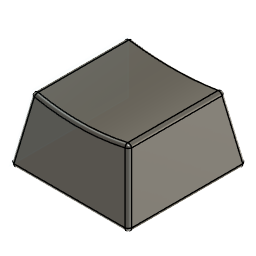
Keycap (Autodesk Fusion 360 design; units mm, degrees)
part number: 2026-06-10-19-01-09-596
Autodesk Fusion 360 part; units mm, degrees
sketch "Sketch1" plane through (0, 0, 0) normal (0, 0, 1) x (1, 0, 0)
  line L0 (9, 9) -> (-9, 9)
  line L1 (-9, 9) -> (-9, -9)
  line L2 (-9, -9) -> (9, -9)
  line L3 (9, -9) -> (9, 9)
  line L4 (9, 9) -> (-9, -9) construction
  line L5 (-9, 9) -> (9, -9) construction
  dimension "d1" = 18
  dimension "d2" = 18
  constraint horizontal L0
  constraint perpendicular L0 L1
  constraint parallel L0 L2
  constraint parallel L1 L3
  constraint coincident L4 origin
  constraint coincident L5 origin
  measures "d1" distance of L0.start L0.end
  measures "d2" distance of L0.start L2.end
extrude "Extrude1" add sketch "Sketch1" along normal blind 10 draft -10
sketch "Sketch2" plane through (-8.7286, 0, 1.5391) normal (-0.984808, 0, 0.173648) x (0, -1, 0)
  line L0 (7.2367, 8.5914) -> (-7.2367, 8.5914)
  line L1 (-7.2367, 8.5914) -> (-9, -1.5628)
  line L2 (-9, -1.5628) -> (9, -1.5628)
  line L3 (9, -1.5628) -> (7.2367, 8.5914)
sketch "Sketch3" plane through (0, 0, 0) normal (0, 1, 0) x (1, 0, 0)
  circle A0 centre (-0.4225, -45.9852) radius 36.7913
  point P0 (7.2367, -10)
  constraint coincident A0 P0
extrude "Extrude2" cut sketch "Sketch3" along normal mid plane 20
sketch "Sketch4" plane through (0, 0, 0) normal (0, 0, 1) x (1, 0, 0)
  line L0 (3, 0.35) -> (3, -0.35)
  line L1 (-3, -0.35) -> (-3, 0.35)
  line L2 (-3, 0.75) -> (3, -0.75) construction
  line L3 (3, 0.75) -> (-3, -0.75) construction
  line L4 (-0.35, 3) -> (0.35, 3)
  line L5 (0.35, -3) -> (-0.35, -3)
  line L6 (-0.75, 3) -> (0.75, -3) construction
  line L7 (0.75, 3) -> (-0.75, -3) construction
  line L8 (-0.75, -2.6) -> (-0.75, -1.15)
  line L9 (-0.75, 1.15) -> (-0.75, 2.6)
  line L10 (2.6, -0.75) -> (1.15, -0.75)
  line L11 (-1.15, -0.75) -> (-2.6, -0.75)
  line L12 (0.75, -1.15) -> (0.75, -2.6)
  line L13 (0.75, 2.6) -> (0.75, 1.15)
  line L14 (-2.6, 0.75) -> (-1.15, 0.75)
  line L15 (1.15, 0.75) -> (2.6, 0.75)
  arc A0 (-1.15, 0.75) -> (-0.75, 1.15) centre (-1.15, 1.15) ccw
  arc A1 (-2.6, 0.75) -> (-3, 0.35) centre (-2.6, 0.35) ccw
  arc A2 (-3, -0.35) -> (-2.6, -0.75) centre (-2.6, -0.35) ccw
  arc A3 (-0.75, -1.15) -> (-1.15, -0.75) centre (-1.15, -1.15) ccw
  arc A4 (-0.75, -2.6) -> (-0.35, -3) centre (-0.35, -2.6) ccw
  arc A5 (0.35, -3) -> (0.75, -2.6) centre (0.35, -2.6) ccw
  arc A6 (1.15, -0.75) -> (0.75, -1.15) centre (1.15, -1.15) ccw
  arc A7 (2.6, -0.75) -> (3, -0.35) centre (2.6, -0.35) ccw
  arc A8 (3, 0.35) -> (2.6, 0.75) centre (2.6, 0.35) ccw
  arc A9 (0.75, 1.15) -> (1.15, 0.75) centre (1.15, 1.15) ccw
  arc A10 (0.75, 2.6) -> (0.35, 3) centre (0.35, 2.6) ccw
  arc A11 (-0.35, 3) -> (-0.75, 2.6) centre (-0.35, 2.6) ccw
  dimension "d9" = 1.5
  dimension "d10" = 1.5
  dimension "d11" = 6
  dimension "d12" = 6
  dimension "d13" = 0.4
  dimension "d14" = 0.4
  dimension "d15" = 0.4
  dimension "d16" = 0.4
  dimension "d17" = 0.4
  dimension "d18" = 0.4
  dimension "d19" = 0.4
  dimension "d20" = 0.4
  dimension "d21" = 0.4
  dimension "d22" = 0.4
  dimension "d23" = 0.4
  dimension "d24" = 0.4
  constraint horizontal L14
  constraint perpendicular L0 L15
  constraint parallel L10 L15
  constraint parallel L0 L1
  constraint coincident L2 origin
  constraint coincident L3 origin
  constraint horizontal L4
  constraint perpendicular L4 L13
  constraint parallel L4 L5
  constraint parallel L8 L12
  constraint coincident L6 origin
  constraint coincident L7 origin
  constraint collinear L8 L9
  constraint collinear L10 L11
  constraint collinear L14 L15
  constraint tangent L9 A0
  constraint tangent L14 A0
  constraint coincident L2.start L14
  constraint coincident L2.start L1
  constraint tangent L14 A1
  constraint tangent L1 A1
  constraint coincident L3.end L11
  constraint coincident L3.end L1
  constraint tangent L11 A2
  constraint tangent L1 A2
  constraint tangent L8 A3
  constraint tangent L11 A3
  constraint coincident L7.end L5
  constraint coincident L7.end L8
  constraint tangent L5 A4
  constraint tangent L8 A4
  constraint coincident L6.end L5
  constraint coincident L6.end L12
  constraint tangent L5 A5
  constraint tangent L12 A5
  constraint tangent L10 A6
  constraint tangent L12 A6
  constraint coincident L2.end L10
  constraint coincident L2.end L0
  constraint tangent L10 A7
  constraint tangent L0 A7
  constraint coincident L3.start L0
  constraint coincident L3.start L15
  constraint tangent L0 A8
  constraint tangent L15 A8
  constraint tangent L15 A9
  constraint tangent L13 A9
  constraint coincident L7.start L13
  constraint coincident L7.start L4
  constraint tangent L13 A10
  constraint tangent L4 A10
  constraint coincident L6.start L4
  constraint coincident L6.start L9
  constraint tangent L4 A11
  constraint tangent L9 A11
  measures "d9" distance of L3.start L2.end
  measures "d10" distance of L6.end L7.end
  measures "d11" distance of L2.start L3.start
  measures "d12" distance of L6.start L7.end
  measures "d13" radius of A0
  measures "d14" radius of A1
  measures "d15" radius of A2
  measures "d16" radius of A3
  measures "d17" radius of A4
  measures "d18" radius of A5
  measures "d19" radius of A6
  measures "d20" radius of A7
  measures "d21" radius of A8
  measures "d22" radius of A9
  measures "d23" radius of A10
  measures "d24" radius of A11
extrude "Extrude3" cut sketch "Sketch4" along normal blind 8
fillet "Fillet2" radius 0.5 60 edges at (-7.2657, 0, 9.8359) (-9, 0, 0) (8.1184, 8.1184, 5) (8.1184, -8.1184, 5) (-8.1328, 8.1328, 4.918) (1.875, 0.75, 0) (0.8672, 0.8672, 0) (0.75, 1.875, 0) (0.6328, 2.8828, 0) (0, 3, 0) (-0.6328, 2.8828, 0) (-0.75, 1.875, 0) (-0.8672, 0.8672, 0) (-1.875, 0.75, 0) (-2.8828, 0.6328, 0) (-3, 0, 0) (-2.8828, -0.6328, 0) (-1.875, -0.75, 0) (-0.8672, -0.8672, 0) (-0.75, -1.875, 0) (-0.6328, -2.8828, 0) (0, -3, 0) (0.6328, -2.8828, 0) (0.75, -1.875, 0) (0.8672, -0.8672, 0) (1.875, -0.75, 0) (2.8828, -0.6328, 0) (3, 0, 0) (2.8828, 0.6328, 0) (0, -9, 0) (0, 9, 0) (7.2367, 0, 10) (-0.0063, -7.3785, 9.1963) (-0.0063, 7.3785, 9.1963) (-8.1328, -8.1328, 4.918) (9, 0, 0) (1.875, 0.75, 8) (0.8672, 0.8672, 8) (0.75, 1.875, 8) (0.6328, 2.8828, 8) (0, 3, 8) (-0.6328, 2.8828, 8) (-0.75, 1.875, 8) (-0.8672, 0.8672, 8) (-1.875, 0.75, 8) (-2.8828, 0.6328, 8) (-3, 0, 8) (-2.8828, -0.6328, 8) (-1.875, -0.75, 8) (-0.8672, -0.8672, 8) (-0.75, -1.875, 8) (-0.6328, -2.8828, 8) (0, -3, 8) (0.6328, -2.8828, 8) (0.75, -1.875, 8) (0.8672, -0.8672, 8) (1.875, -0.75, 8) (2.8828, -0.6328, 8) (3, 0, 8) (2.8828, 0.6328, 8) 31 faces at (-8.4219, 2.4219, 3.2786) (-0.8128, -8.4564, 3.0831) (8.4122, -2.4122, 3.3333) (0.75, 2.1167, 5.3333) (1.0557, 0.7613, 5.3333) (1.6333, 0.75, 2.6667) (2.9144, 0.5973, 5.3333) (3, 0.1167, 2.6667) (2.832, -0.6758, 5.3333) (2.1167, -0.75, 2.6667) (0.8605, -0.874, 5.3333) (0.75, -1.6333, 2.6667) (0.6758, -2.832, 5.3333) (0.1167, -3, 2.6667) (-0.626, -2.8895, 5.3333) (-0.75, -2.1167, 2.6667) (-0.8036, -0.95, 5.3333) (-1.6333, -0.75, 5.3333) (-2.876, -0.6395, 5.3333) (-3, -0.1167, 2.6667) (-2.8895, 0.626, 5.3333) (-2.1167, 0.75, 5.3333) (-1.0013, 0.7787, 5.3333) (-0.75, 1.6333, 5.3333) (-0.6758, 2.832, 5.3333) (-0.1167, 3, 2.6667) (0.6644, 2.8473, 5.3333) (0.2826, -0.296, 8) (-0.1167, 7, 0) (4.038, -2.4122, 9.4653) (-0.8128, 8.4564, 3.0831)
